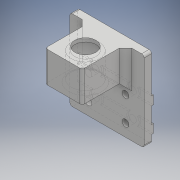
# Autodesk Inventor part: Estrutura - Suporte Rolamento Z Motor
Saved by Autodesk Inventor 2017 (Build 210142000, 142)
## iProperties
Created: 2020-08-03
Part Number: Estrutura - Suporte Rolamento Z Motor
Material: Generic
Document SubType Name: Modeling
Designer: ale
Density: 1 g/cm^3
Appearance: Default
Author: ale
Autodesk Inventor part; units mm, degrees
ref_plane "YZ Plane" through (0, 0, 0) normal (1, 0, 0) x (0, 1, 0)
ref_plane "XZ Plane" through (0, 0, 0) normal (0, 1, 0) x (-1, 0, 0)
ref_plane "XY Plane" through (0, 0, 0) normal (0, 0, 1) x (1, 0, 0)
sketch "Sketch1" plane through (0, 0, 0) normal (0, 0, 1) x (1, 0, 0)
  circle A0 centre (0, 0) radius 11.4
  line L0 (-15, 17.5) -> (15, 17.5)
  line L1 (15, 17.5) -> (15, -17.5)
  line L2 (15, -17.5) -> (-15, -17.5)
  line L3 (-15, -17.5) -> (-15, 17.5)
  line L4 (-15, 17.5) -> (15, -17.5) construction
  line L5 (15, 17.5) -> (-15, -17.5) construction
  dimension "d0" = 22.8
  dimension "d1" = 30
  dimension "d2" = 35
  constraints: 12 end point, 2 midpoint, 2 parallel, 1 centre point, 1 coincident, 1 horizontal, 1 perpendicular
  measures "d0" diameter of A0
  measures "d1" distance of L1.end L2.end
  measures "d2" distance of L0.end L1.end
extrude "Extrusion1" add sketch "Sketch1" along normal blind 25
sketch "Sketch3" plane through (-15, 17.5, 0) normal (0, 1, 0) x (1, 0, 0)
  line L0 (30, 0) -> (0, 0) projected
  line L1 (0, 0) -> (30, -25)
  line L2 (45, 40) -> (-15, 40)
  line L3 (-15, 40) -> (-15, -25)
  line L4 (-15, -25) -> (45, -25)
  line L5 (45, -25) -> (45, 40)
  line L6 (0, 0) -> (30, 0) projected
  line L7 (30, 0) -> (45, 0)
  line L8 (30, -25) -> (0, -25) projected
  point P0 (15, 0)
  point P1 (15, -12.5)
  dimension "d8" = 60
  dimension "d9" = 65
  dimension "d27" = 0
  constraints: 12 end point, 2 parallel, 1 horizontal, 1 midpoint, 1 perpendicular, 1 point on line
  measures "d8" distance of L4.end L3.end
  measures "d9" distance of L3.end L2.end
  measures "d27" distance between parallel lines of L4 L8
extrude "Extrusion3" add sketch "Sketch3" along normal blind 6
sketch "Sketch4" plane through (-15, 23.5, 0) normal (0, 1, 0) x (1, 0, 0)
  line L0 (-15, 40) -> (-15, -25) projected
  line L1 (45, -25) -> (45, 40) projected
  line L2 (-15, 33.5) -> (45, 33.5)
  line L3 (-15, 26.5) -> (45, 26.5)
  line L4 (-15, 13.5) -> (45, 13.5)
  line L5 (-15, 6.5) -> (45, 6.5)
  line L6 (45, 33.5) -> (45, 26.5)
  line L7 (45, 13.5) -> (45, 6.5)
  line L8 (-15, 6.5) -> (-15, 13.5)
  line L9 (-15, 26.5) -> (-15, 33.5)
  line L10 (45, 40) -> (-15, 40) projected
  dimension "d20" = 6.5
  dimension "d21" = 13.5
  dimension "d22" = 26.5
  dimension "d23" = 33.5
  constraints: 16 end point, 2 collinear, 2 perpendicular
  measures "d20" distance from line of L1.end L2
  measures "d21" distance between parallel lines of L10 L3
  measures "d22" distance between parallel lines of L4 L10
  measures "d23" distance between parallel lines of L5 L10
extrude "Extrusion4" add sketch "Sketch4" along normal blind 1.5 contours L2 L1 L3 L0 | L4 L1 L5 L0
sketch "Sketch5" plane through (0, 0, 25) normal (0, 0, 1) x (1, 0, 0)
  circle A0 centre (0, 0) radius 11.4
  circle A1 centre (0, 0) radius 8.5
  dimension "d24" = 17
  constraints: 2 centre point, 2 coincident
  measures "d24" diameter of A1
extrude "Extrusion5" add sketch "Sketch5" against normal blind 3
fillet "Fillet1" radius 2 7 edges at (15, -17.5, 12.5) (-15, -17.5, 12.5) (-30, 20.5, -40) (30, 20.5, -40) (30, 20.5, 25) (-30, 20.5, 25) (-11.4, 0, 0)
chamfer "Chamfer1" distance 5 angle 45 3 edges at (15, 17.5, 12.5) (-15, 17.5, 12.5) (0, 17.5, 0)
sketch "Sketch6" plane through (-15, 25, 0) normal (0, 1, 0) x (1, 0, 0)
  line L0 (43, 40) -> (-13, 40) projected
  line L1 (0, 33.5) -> (0, 26.5)
  line L2 (30, 33.5) -> (30, 26.5)
  line L3 (-15, 33.5) -> (-15, 26.5) projected
  line L4 (-15, 26.5) -> (45, 26.5) projected
  line L5 (45, 33.5) -> (-15, 33.5) projected
  line L6 (-15, 33.5) -> (45, 33.5)
  line L7 (0, 30) -> (30, 30)
  line L8 (-15, 13.5) -> (45, 13.5) projected
  line L9 (-15, 26.5) -> (-15, 13.5)
  line L10 (-15, 26.5) -> (-15, 13.5) projected
  line L11 (-15, 20) -> (45, 20)
  point P0 (15, 0)
  point P1 (0, 10)
  point P2 (30, 10)
  constraints: 12 end point, 4 point on line, 3 midpoint, 2 coincident, 2 perpendicular, 2 symmetric about line, 1 collinear
hole "Hole1" at (-15, 25, -30) at (15, 25, -30) at (-15, 25, -10) at (15, 25, -10) direction (0, -1, 0) diameter 5.5 end through all counterbore diameter 10 counterbore depth 1.5
body "Solid1"
